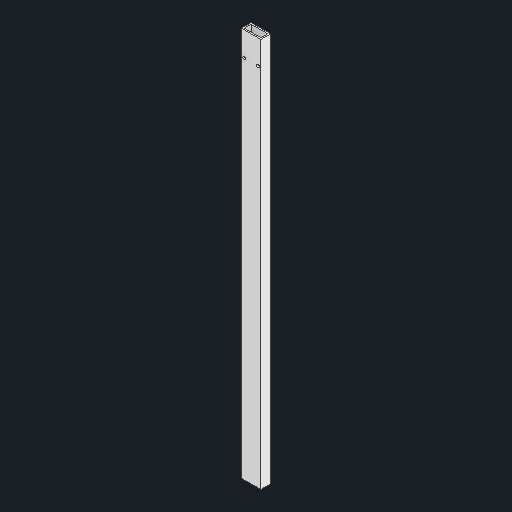
# Autodesk Inventor part: tibea_profile
Saved by Autodesk Inventor 2026 (Build 300175000, 175)
## iProperties
Created: 2026-04-23
Part Number: tibea_profile
Material: Алюминий
Document SubType Name: Modeling
Designer: user
Density: 2.7 g/cm^3
Appearance: Белый
Mass: 698.893 g
Surface Area: 1734.44 cm^2
Volume: 258.849 cm^3
Author: user
Autodesk Inventor part; units mm, degrees
ref_plane "YZ Plane" through (0, 0, 0) normal (1, 0, 0) x (0, 1, 0)
ref_plane "XZ Plane" through (0, 0, 0) normal (0, 1, 0) x (-1, 0, 0)
ref_plane "XY Plane" through (0, 0, 0) normal (0, 0, 1) x (1, 0, 0)
sketch "Эскиз1" plane through (0, 0, 0) normal (0, 1, 0) x (-1, 0, 0)
  line L0 (0, 0) -> (40, 0)
  line L1 (40, 0) -> (40, -20)
  line L2 (40, -20) -> (0, -20)
  line L3 (0, -20) -> (0, 0)
  line L4 (37, -3) -> (3, -3)
  line L5 (3, -3) -> (3, -17)
  line L6 (3, -17) -> (37, -17)
  line L7 (37, -17) -> (37, -3)
  dimension "d0" = 20
  dimension "d1" = 40
  dimension "d2" = 3
  constraints: 16 end point, 4 parallel, 2 perpendicular, 1 horizontal, 3 other
  measures "d0" distance of L0.end L1.end
  measures "d1" distance of L1.end L2.end
  measures "d2" distance between parallel lines of L0 L4
extrude "Выдавливание1" add sketch "Эскиз1" along normal blind 800
sketch "Эскиз2" plane through (-40, 0, 0) normal (0, 0, 1) x (1, 0, 0)
  circle A0 centre (6.05, 750) radius 3.05
  line L0 (3, 0) -> (3, 800) projected
  line L1 (0, 800) -> (40, 800) projected
  line L2 (20, 819.3664) -> (20, 691.613)
  circle A1 centre (33.95, 750) radius 3.05
  point P0 (40, 0)
  dimension "d5" = 50
  dimension "d6" = 6.1
  constraints: 2 centre point, 2 end point, 1 symmetric about line, 1 tangent, 1 vertical, 1 other
  measures "d5" distance from line of L1 A0.centre
  measures "d6" diameter of A0
extrude "Выдавливание2" cut sketch "Эскиз2" against normal through all
equation "\"d0\" = width_profile_tibea"
equation "\"d1\" = hight_profile_tibea"
equation "\"d2\" = thickness_profile_tibea"
equation "\"d3\" = length_profile_tibia"
equation "\"d6\" = d_main_screw_holes"
equation "\"width_profile_tibea\" = 20"
equation "\"hight_profile_tibea\" = 40"
equation "\"length_profile_tibia\" = 800"
equation "\"thickness_profile_tibea\" = 3"
equation "\"tolerance_plazma\" = 0.1"
equation "\"d_main_screw_holes\" = 6.1"
equation "\"thickness_steel\" = 3"
equation "\"hight_shaft_shift\" = 37"
equation "\"thickness_profile_femur\" = 3"
equation "\"width_shaft_shift\" = 35"
equation "\"width_flattened_surface\" = 12"
